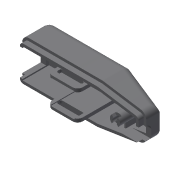
# Autodesk Inventor part: enctop
Saved by Autodesk Inventor 2022 Beta2 (Build 260130000, 130) ContinuousBuild 0
## iProperties
Shininess: 64.0
Length Units: 11269
Angle Units: 11279
Time Units: 11290
Mass Units: 11283
Length Display Precision: 3
Angle Display Precision: 2
Created: 2002-02-13
Part Number: enctop
Document SubType Name: Modeling
Designer: Administrator
Density: 1 g/cm^3
Material: Generic
Appearance: Light Gray
Density: 0.0
Volumn: 0.0
Area: 0.0
PropertySet Name: Model Information
Control State: 0
Master: False
Checked Out: False
Last Check In By: PMILLER
Last Check In Date: 2007-04-03
Author: Administrator
Autodesk Inventor part; units mm, degrees
sketch "Sketch1" plane through (0, 0, 0) normal (0, 0, 1) x (1, 0, 0)
  line L0 (8.2169, 11.6469) -> (8.2169, -7.4031)
  line L1 (8.2169, -7.4031) -> (46.3169, -7.4031)
  line L2 (46.3169, -7.4031) -> (66.9544, -4.2281)
  line L3 (66.9544, -4.2281) -> (66.9544, 8.4719)
  line L4 (66.9544, 8.4719) -> (46.3169, 11.6469)
  line L5 (46.3169, 11.6469) -> (8.2169, 11.6469)
  line L6 (66.9544, 2.1219) -> (8.2169, 2.1219) construction
  dimension "d0" = 19.05
  dimension "d1" = 38.1
  dimension "d2" = 58.7375
  dimension "d3" = 12.7
  constraints: 14 end point, 2 equal length, 2 midpoint, 2 parallel, 1 horizontal, 1 perpendicular, 1 vertical
  measures "d0" distance of L0.start L0.end
  measures "d1" distance of L4.end L0.start
  measures "d2" horizontal distance of L3.end L0.start
  measures "d3" distance of L2.end L3.end
extrude "Extrusion1" add sketch "Sketch1" along normal blind 12.7
sketch "Sketch2" plane through (8.2169, -7.4031, 0) normal (0, -1, 0) x (1, 0, 0)
  line L0 (38.1, 0) -> (38.1, 12.7) projected
  line L1 (38.1, 0) -> (58.7375, 0)
  line L2 (58.7375, 0) -> (58.7375, 6.35)
  line L3 (58.7375, 6.35) -> (38.1, 0)
  line L4 (58.7375, 12.7) -> (38.1, 12.7) projected
  line L5 (58.7375, 0) -> (58.7375, 12.7) projected
  dimension "d6" = 6.35
  constraints: 6 end point, 2 perpendicular, 1 collinear
  measures "d6" distance from line of L4 L2.end
extrude "Extrusion2" cut sketch "Sketch2" against normal through all contours L3 L2 L1
shell "Shell1" thickness 2.54 removed faces 1 at (20.9169, -1.0531, 12.7)
sketch "Sketch3" plane through (0, 0, 12.7) normal (0, 0, 1) x (1, 0, 0)
  line L0 (64.4144, 6.2927) -> (64.4144, -2.049) projected
  line L1 (64.4144, -2.049) -> (46.1226, -4.8631) projected
  line L2 (46.1226, -4.8631) -> (10.7569, -4.8631) projected
  line L3 (10.7569, -4.8631) -> (10.7569, 9.1069) projected
  line L4 (10.7569, 9.1069) -> (46.1226, 9.1069) projected
  line L5 (46.1226, 9.1069) -> (64.4144, 6.2927) projected
  line L6 (66.9544, -4.2281) -> (46.3169, -7.4031) projected
  line L7 (66.9544, 8.4719) -> (66.9544, -4.2281) projected
  line L8 (9.4869, 10.3769) -> (46.2197, 10.3769)
  line L9 (46.2197, 10.3769) -> (65.6844, 7.3823)
  line L10 (65.6844, 7.3823) -> (65.6844, -3.1386)
  line L11 (65.6844, -3.1386) -> (46.2197, -6.1331)
  line L12 (46.2197, -6.1331) -> (9.4869, -6.1331)
  line L13 (9.4869, -6.1331) -> (9.4869, 10.3769)
  dimension "d10" = 1.27
  dimension "d11" = 1.27
  dimension "d12" = 1.27
  dimension "d13" = 1.27
  dimension "d14" = 1.27
  constraints: 12 end point, 4 parallel, 3 perpendicular
  measures "d10" horizontal distance of L3.end L8.start
  measures "d11" horizontal distance of L2.end L12.end
  measures "d12" horizontal distance of L9.end L0.start
  measures "d13" distance between parallel lines of L9 L5
  measures "d14" distance from line of L0.end L11
extrude "Extrusion3" add sketch "Sketch3" along normal blind 2.3813
fillet "Fillet1" radius 3.175 11 edges at (8.2169, 11.6469, 6.35) (8.2169, -7.4031, 6.35) (8.2169, 2.1219, 0) (27.2669, -7.4031, 0) (46.3169, -7.4031, 6.35) (56.6356, -5.8156, 3.175) (66.9544, -4.2281, 9.525) (27.2669, 11.6469, 0) (46.3169, 11.6469, 6.35) (56.6356, 10.0594, 3.175) (66.9544, 8.4719, 9.525)
fillet "Fillet2" radius 1.5875 4 edges at (9.4869, 10.3769, 13.8906) (9.4869, -6.1331, 13.8906) (65.6844, 7.3823, 13.8906) (65.6844, -3.1386, 13.8906)
ref_plane "Work Plane1" through (23.4569, -4.8631, 2.54) normal (1, 0, 0) x (0, 0, -1)
sketch "Sketch4" plane through (66.9544, -1.5043, 12.7) normal (1, 0, 0) x (0, 0, -1)
  line L0 (6.35, 0.3448) -> (6.35, 6.9074) projected
  line L1 (0, 4.7994) -> (-2.3812, 4.7994)
  line L2 (-2.3812, 4.7994) -> (-2.3813, -1.5506)
  line L3 (-2.3813, -1.5506) -> (2.3812, -1.5506)
  line L4 (2.3812, -1.5506) -> (2.3812, 2.4182)
  arc A0 (2.3812, 2.4182) -> (0, 4.7994) centre (0, 2.4182) ccw
  line L5 (0, -3.1381) -> (4.005, -3.1381) projected
  line L6 (-2.3812, 7.5246) -> (-2.3812, -0.2724) projected
  dimension "d19" = 2.3813
  dimension "d20" = 6.35
  dimension "d21" = 4.7625
  dimension "d22" = 1.5875
  constraints: 8 end point, 2 perpendicular, 2 point on circle, 2 tangent, 1 centre point, 1 collinear, 1 parallel, 1 vertical
  measures "d19" radius of A0
  measures "d20" distance of L1.end L2.end
  measures "d21" distance of L2.end L3.end
  measures "d22" distance between parallel lines of L5 L3
extrude "Extrusion4" cut sketch "Sketch4" against normal up to surface (43.4975 mm away)
sketch "Sketch5" plane through (8.2169, -4.2281, 3.175) normal (-1, 0, 0) x (0, 0, 1)
  line L0 (0, 12.7) -> (9.525, 12.7) projected
  line L1 (0.7937, 12.7) -> (11.9062, 12.7)
  line L2 (11.9062, 12.7) -> (11.9062, 0)
  line L3 (11.9062, 0) -> (0.7937, 0)
  line L4 (0.7937, 0) -> (0.7937, 12.7)
  line L5 (11.9062, -0.3175) -> (11.9062, 13.0175) projected
  dimension "d26" = 11.1125
  constraints: 8 end point, 2 collinear, 2 parallel, 1 horizontal, 1 perpendicular
  measures "d26" distance of L2.end L3.end
extrude "Extrusion5" cut sketch "Sketch5" against normal up to surface (15.24 mm away)
ref_plane "Work Plane2" through (0, 0, 11.9062) normal (0, 0, 1) x (1, 0, 0)
sketch "Sketch6" plane through (0, 0, 11.9062) normal (0, 0, 1) x (1, 0, 0)
  line L0 (55.6831, 7.636) -> (55.6831, -3.3923)
  line L1 (56.4769, 7.5139) -> (56.4769, -3.2702)
  line L2 (64.4144, -2.049) -> (64.4144, 0.9139) projected
  line L3 (57.8767, -3.0548) -> (46.1226, -4.8631) projected
  line L4 (46.1226, 9.1069) -> (64.4144, 6.2927) projected
  line L5 (55.6831, -3.3923) -> (56.4769, -3.2702)
  line L6 (56.4769, 7.5139) -> (55.6831, 7.636)
  dimension "d31" = 0.7937
  dimension "d32" = 7.9375
  constraints: 8 end point, 2 collinear, 1 parallel, 1 vertical
  measures "d31" distance between parallel lines of L1 L0
  measures "d32" distance between parallel lines of L2 L1
extrude "Extrusion6" add sketch "Sketch6" against normal up to next
ref_plane "Work Plane3" through (0, 0, 16.6687) normal (0, 0, 1) x (1, 0, 0)
sketch "Sketch7" plane through (0, 0, 16.6687) normal (0, 0, 1) x (1, 0, 0)
  circle A0 centre (56.08, 2.1219) radius 2.3813
  circle A1 centre (56.08, 2.1219) radius 5.3897 construction
  circle A2 centre (56.08, 2.1219) radius 0.3969 construction
  line L0 (57.8767, -3.0548) -> (46.1226, -4.8631) projected
  line L1 (46.1226, 9.1069) -> (64.4144, 6.2927) projected
  line L2 (56.4769, -3.2702) -> (56.4769, 7.5139) projected
  line L3 (55.6831, 7.636) -> (55.6831, -3.3923) projected
  dimension "d36" = 4.7625
  constraints: 4 tangent, 3 centre point, 2 coincident
  measures "d36" diameter of A0
extrude "Extrusion7" add sketch "Sketch7" against normal up to surface contours A0 L2 | L2 A0 L3 | L3 A0 surface through (66.2074, -7.4031, 8.7777) normal (-0.2940858, 0, 0.955779)
sketch "Sketch8" plane through (56.08, 2.1219, 16.6687) normal (0, 0, 1) x (1, 0, 0)
  circle A0 centre (0, 0) radius 2.3813 projected
  circle A1 centre (0, 0) radius 1.27
  dimension "d39" = 2.54
  constraints: 1 centre point, 1 coincident
  measures "d39" diameter of A1
extrude "Extrusion8" cut sketch "Sketch8" against normal up to surface contours A1 surface through (66.2074, -7.4031, 8.7777) normal (-0.2940858, 0, 0.955779)
sketch "Sketch9" plane through (56.08, 2.1219, 16.6687) normal (0, 0, 1) x (1, 0, 0)
  circle A0 centre (0, 0) radius 2.3813 projected
  line L0 (0, 0) -> (1.9981, 2.3813)
  line L1 (1.9981, 2.3813) -> (-1.9981, 2.3813)
  line L2 (-1.9981, 2.3813) -> (0, 0)
  dimension "d42" = 80
  constraints: 6 end point, 1 equal length, 1 horizontal, 1 tangent
  measures "d42" angle of L2 L0
extrude "Extrusion9" cut sketch "Sketch9" against normal blind 1.5875 contours L0 L2 A0 | A0 L1 L0 | L2 L1 A0 picked at (0.1831, 1.5661)
pattern_circular "Circular Pattern1" count 2 over 360 about axis through (56.08, 2.1219, 16.6687) along (0, 0, -1) of "Extrusion9"
sketch "Sketch10" plane through (10.7569, -4.8631, 2.54) normal (0, 0, 1) x (1, 0, 0)
  line L0 (0, 13.97) -> (0, 0) projected
  line L1 (16.6688, 13.97) -> (30.9563, 13.97)
  line L2 (30.9563, 13.97) -> (30.9563, 12.3825)
  line L3 (16.6688, 12.3825) -> (16.6688, 13.97)
  line L4 (0, 13.97) -> (35.3658, 13.97) projected
  line L5 (16.6688, 12.3825) -> (18.2563, 12.3825)
  line L6 (18.2563, 12.7794) -> (29.3688, 12.7794)
  line L7 (29.3688, 12.7794) -> (29.3688, 12.3825)
  line L8 (29.3688, 12.3825) -> (30.9563, 12.3825)
  line L9 (18.2563, 12.7794) -> (18.2563, 12.3825)
  dimension "d48" = 1.5875
  dimension "d49" = 14.2875
  dimension "d50" = 16.6687
  dimension "d53" = 1.5875
  dimension "d54" = 0.3969
  constraints: 16 end point, 4 perpendicular, 3 collinear, 3 parallel, 1 horizontal
  measures "d48" distance of L3.start L1.start
  measures "d49" distance of L2.end L3.start
  measures "d50" distance from line of L1.start L0
  measures "d53" distance of L3.start L5.end
  measures "d54" distance of L5.end L6.start
extrude "Extrusion10" add sketch "Sketch10" along normal blind 17.4625
ref_plane "Work Plane4" through (56.08, 2.1219, 16.6687) normal (0, -1, 0) x (1, 0, 0)
fillet "Fillet3" radius 2.3813 2 edges at (27.4256, 8.3131, 20.0025) (41.7131, 8.3131, 20.0025)
sketch "Sketch11" plane through (29.0131, 7.9162, 2.54) normal (0, -1, 0) x (1, 0, 0)
  line L0 (10.3188, 17.4625) -> (0.7938, 17.4625) projected
  line L1 (0, 0) -> (0, 17.3263) projected
  line L2 (11.1125, 0) -> (11.1125, 17.3263) projected
  line L3 (0.7937, 14.9225) -> (10.3188, 14.9225)
  line L4 (11.1125, 14.1288) -> (11.1125, 13.335)
  line L5 (10.3188, 12.5413) -> (0.7937, 12.5413)
  line L6 (0, 13.335) -> (0, 14.1288)
  arc A0 (11.1125, 14.1288) -> (10.3188, 14.9225) centre (10.3188, 14.1288) ccw
  arc A1 (0.7937, 14.9225) -> (0, 14.1288) centre (0.7937, 14.1288) ccw
  arc A2 (0, 13.335) -> (0.7937, 12.5413) centre (0.7937, 13.335) ccw
  arc A3 (10.3188, 12.5413) -> (11.1125, 13.335) centre (10.3188, 13.335) ccw
  dimension "d58" = 0.7937
  dimension "d59" = 2.54
  dimension "d60" = 2.3813
  constraints: 8 end point, 8 point on circle, 8 tangent, 4 centre point, 3 equal radius, 2 collinear, 2 parallel, 1 horizontal, 1 perpendicular
  measures "d58" radius of A0
  measures "d59" distance between parallel lines of L3 L0
  measures "d60" distance between parallel lines of L5 L3
extrude "Extrusion11" cut sketch "Sketch11" against normal through all
mirror "Mirror1" about plane through (56.08, 2.1219, 16.6687) normal (0, -1, 0) of "Extrusion10", "Extrusion11", "Fillet3"
body "Solid1"
